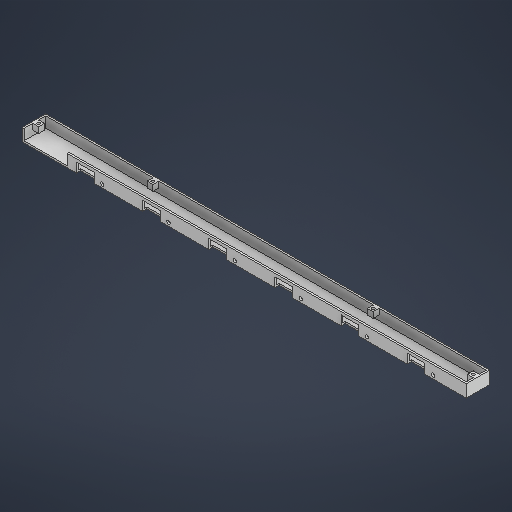
# Autodesk Inventor part: PCB_Kabelkanal_1.0
Saved by Autodesk Inventor 2027 (Build 310192060, 192F)
## iProperties
Created: 2026-05-05
Part Number: PCB_Kabelkanal_1.0
Material: Generisch
Document SubType Name: Modeling
Designer: simon
Density: 1 g/cm^3
Appearance: Vorgabe
Author: simon
Autodesk Inventor part; units mm, degrees
ref_plane "YZ Plane" through (0, 0, 0) normal (1, 0, 0) x (0, 1, 0)
ref_plane "XZ Plane" through (0, 0, 0) normal (0, 1, 0) x (-1, 0, 0)
ref_plane "XY Plane" through (0, 0, 0) normal (0, 0, 1) x (1, 0, 0)
sketch "Skizze1" plane through (0, 0, 0) normal (0, 0, 1) x (1, 0, 0)
  line L0 (-188.78, 10) -> (188.78, 10)
  line L1 (188.78, 10) -> (188.78, -10)
  line L2 (188.78, -10) -> (-188.78, -10)
  line L3 (-188.78, -10) -> (-188.78, 10)
  line L4 (-264.292, 0) -> (264.292, 0) construction
  line L5 (0, -14) -> (0, 14) construction
  point P0 (0, 0)
  dimension "d0" = 377.56
  dimension "d1" = 20
  constraints: 8 end point, 2 parallel, 1 horizontal, 1 perpendicular, 2 other
  measures "d0" distance of L0.start L0.end
  measures "d1" distance between parallel lines of L0 L2
extrude "Extrusion1" add sketch "Skizze1" along normal blind 10.6
sketch "Skizze2" plane through (0, 0, 10.6) normal (0, 0, 1) x (1, 0, 0)
  line L0 (-187.28, 8.5) -> (187.28, 8.5)
  line L1 (187.28, 8.5) -> (187.28, -8.5)
  line L2 (187.28, -8.5) -> (-187.28, -8.5)
  line L3 (-187.28, -8.5) -> (-187.28, 8.5)
  line L4 (-264.292, 0) -> (264.292, 0) construction
  line L5 (0, -14) -> (0, 14) construction
  line L6 (-188.78, -10) -> (188.78, -10) construction
  line L7 (188.78, -10) -> (188.78, 10) construction
  point P0 (0, 0)
  dimension "d4" = 1.5
  dimension "d5" = 1.5
  constraints: 8 end point, 2 parallel, 1 horizontal, 1 perpendicular, 2 other
  measures "d4" distance between parallel lines of L7 L1
  measures "d5" distance between parallel lines of L6 L2
extrude "Extrusion2" cut sketch "Skizze2" against normal blind 9.1
sketch "Skizze3" plane through (-188.78, -10, 0) normal (0, -1, 0) x (1, 0, 0)
  line L0 (0, 0) -> (377.56, 0) projected
  line L1 (377.56, 0) -> (377.56, 10.6) projected
  line L2 (0, 10.6) -> (377.56, 10.6) projected
  line L3 (0, 0) -> (0, 10.6) projected
  point P0 (188.78, 0)
  point P1 (349.43, 3)
  dimension "d9" = 28.13
  dimension "d10" = 3
  measures "d9" distance from line of L1 point (349.43, 3)
  measures "d10" distance from line of L0 point (349.43, 3)
hole "Bohrung1" at (160.65, -10, 3) direction (0, 1, 0) diameter 3 depth 1.5
pattern_linear "Rechteckige Anordnung1" count 6 spacing 56.26 along (-1, 0, 0) of "Bohrung1"
sketch "Skizze4" plane through (-188.78, -10, 0) normal (0, -1, 0) x (1, 0, 0)
  circle A0 centre (68.13, 3) radius 1.5 projected
  circle A1 centre (124.39, 3) radius 1.5 projected
  circle A2 centre (180.65, 3) radius 1.5 projected
  circle A3 centre (236.91, 3) radius 1.5 projected
  circle A4 centre (293.17, 3) radius 1.5 projected
  circle A5 centre (349.43, 3) radius 1.5 projected
  line L0 (0, 0) -> (377.56, 0) projected
  line L1 (377.56, 0) -> (377.56, 10.6) projected
  line L2 (0, 10.6) -> (377.56, 10.6) projected
  line L3 (0, 0) -> (0, 10.6) projected
  line L4 (38.5, 10.6) -> (38.5, 0) construction
  line L5 (1.5, 10.6) -> (1.5, 1.5) projected
  line L6 (38.5, 1.5) -> (1.5, 1.5)
  line L7 (1.5, 1.5) -> (1.5, 10.6)
  line L8 (1.5, 10.6) -> (38.5, 10.6)
  line L9 (38.5, 10.6) -> (38.5, 1.5)
  point P0 (188.78, 0)
  dimension "d21" = 29.63
  constraints: 10 end point, 3 point on line, 2 parallel, 2 perpendicular, 1 horizontal, 1 tangent
  measures "d21" distance from line of A0.centre L4
extrude "Extrusion3" cut sketch "Skizze4" against normal up to surface (1.5 mm away) contours L2 L9 L6 L5
sketch "Skizze5" plane through (-188.78, -10, 0) normal (0, -1, 0) x (1, 0, 0)
  line L0 (0, 0) -> (377.56, 0) projected
  line L1 (342.43, 0) -> (327.43, 0)
  line L2 (327.43, 0) -> (327.43, 8.1)
  line L3 (327.43, 8.1) -> (342.43, 8.1)
  line L4 (342.43, 8.1) -> (342.43, 0)
  line L5 (38.5, 10.6) -> (377.56, 10.6) projected
  line L6 (377.56, 0) -> (377.56, 10.6) projected
  circle A0 centre (349.43, 3) radius 1.5 projected
  point P0 (188.78, 0)
  point P1 (327.43, 0)
  dimension "d24" = 15
  dimension "d25" = 2.5
  dimension "d27" = 7
  constraints: 8 end point, 2 parallel, 1 horizontal, 1 perpendicular, 1 point on line
  measures "d24" distance of L2.end L3.end
  measures "d25" distance between parallel lines of L5 L3
  measures "d27" distance from line of A0.centre L4
extrude "Extrusion4" cut sketch "Skizze5" against normal blind 3.5 contours L2 L3 L4 L0
pattern_linear "Rechteckige Anordnung2" count 6 spacing 56.26 along (-1, 0, 0) of "Extrusion4"
sketch "Skizze7" plane through (0, 0, 10.6) normal (0, 0, 1) x (1, 0, 0)
  line L0 (-187.28, -10) -> (-187.28, 8.5) projected
  line L1 (-187.28, -2.5) -> (-182.28, -2.5)
  line L2 (-182.28, -2.5) -> (-182.28, 2.5)
  line L3 (-182.28, 2.5) -> (-187.28, 2.5)
  line L4 (-187.28, 2.5) -> (-187.28, -2.5)
  line L5 (-264.292, 0) -> (264.292, 0) construction
  line L6 (0, -14) -> (0, 14) projected
  line L7 (-187.28, 8.5) -> (187.28, 8.5) projected
  line L8 (-96.14, 8.5) -> (-91.14, 8.5)
  line L9 (-91.14, 8.5) -> (-91.14, 3.5)
  line L10 (-91.14, 3.5) -> (-96.14, 3.5)
  line L11 (-96.14, 3.5) -> (-96.14, 8.5)
  circle A0 centre (-184.78, 0) radius 1.25
  circle A1 centre (-93.64, 6) radius 1.25
  point P0 (0, 0)
  dimension "d36" = 5
  dimension "d37" = 5
  dimension "d38" = 5
  dimension "d39" = 5
  dimension "d40" = 91.14
  dimension "d41" = 91.14
  dimension "d42" = 2.5
  dimension "d43" = 2.5
  dimension "d44" = 93.64
  dimension "d45" = 6
  dimension "d46" = 184.78
  constraints: 16 end point, 4 parallel, 3 point on line, 2 centre point, 2 horizontal, 2 perpendicular, 1 other
  measures "d36" distance of L3.end L2.end
  measures "d37" distance of L2.end L1.end
  measures "d38" distance of L9.end L10.end
  measures "d39" distance of L8.end L9.end
  measures "d40" distance between parallel lines of L6 L9
  measures "d41" distance between parallel lines of L0 L11
  measures "d42" diameter of A0
  measures "d43" diameter of A1
  measures "d44" distance from line of A1.centre L6
  measures "d45" distance from line of A1.centre L5
  measures "d46" distance from line of A0.centre L6
extrude "Extrusion6" add sketch "Skizze7" against normal blind 5
mirror "Spiegeln2" about plane through (0, 0, 0) normal (1, 0, 0) of "Extrusion6"
